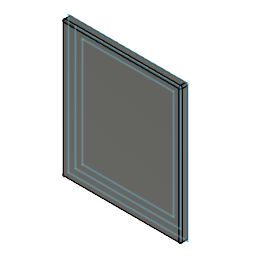
TA-couvercle-V1 (Autodesk Fusion 360 design; units mm, degrees)
part number: 2025-12-22-10-51-43-779
Autodesk Fusion 360 part; units mm, degrees
sketch "Esquisse1" plane through (0, 0, 0) normal (0, 1, 0) x (1, 0, 0)
  line L0 (-10, 10) -> (24, 10)
  line L1 (24, 10) -> (24, -29)
  line L2 (24, -29) -> (-10, -29)
  line L3 (-10, -29) -> (-10, 10)
  line L4 (-8, -27) -> (22, -27)
  line L5 (22, -27) -> (22, 8)
  line L6 (22, 8) -> (-8, 8)
  line L7 (-8, 8) -> (-8, -27)
  line L8 (-6, -25) -> (20, -25)
  line L9 (20, -25) -> (20, 6)
  line L10 (20, 6) -> (-6, 6)
  line L11 (-6, 6) -> (-6, -25)
  constraint horizontal L0
  constraint vertical L1
  constraint horizontal L2
  constraint vertical L3
  constraint horizontal L4
  constraint vertical L5
  constraint horizontal L6
  constraint vertical L7
  constraint horizontal L8
  constraint vertical L9
  constraint horizontal L10
  constraint vertical L11
extrude "Extrusion1" add sketch "Esquisse1" against normal blind 2 contours L0 L1 L2 L3 | L4 L5 L6 L7 | L8 L9 L10 L11 makes body 1
extrude "Extrusion2" add sketch "Esquisse1" along normal blind 2 separate body contours L4 L5 L6 L7 makes body 2
fillet "Congé1" radius 0.5 1 edges at (-10, -1, -10) on bodies 1
fillet "Congé2" radius 0.5 1 edges at (24, -1, -10) on bodies 1
fillet "Congé3" radius 0.5 1 edges at (24, -1, 29) on bodies 1
fillet "Congé4" radius 0.5 1 edges at (-10, -1, 29) on bodies 1
fillet "Congé5" radius 0.5 8 edges at (-9.8536, -2, 28.8536) (-10, -2, 9.5) (-9.8536, -2, -9.8536) (7, -2, -10) (23.8536, -2, -9.8536) (24, -2, 9.5) (23.8536, -2, 28.8536) (7, -2, 29) on bodies 1
